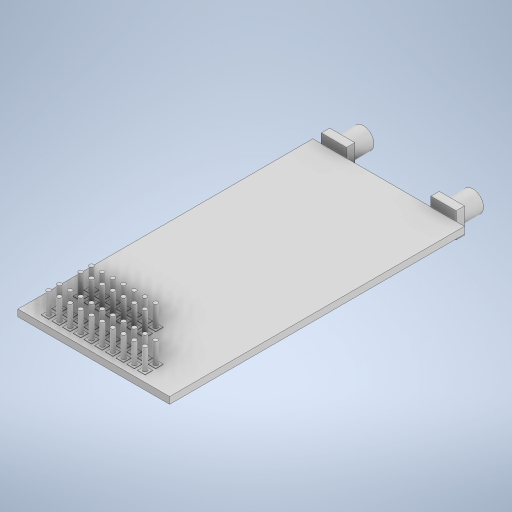
# Autodesk Inventor part: LoRa_board
Saved by Autodesk Inventor 2023 (Build 270158000, 158)
## iProperties
Created: 2023-03-23
Part Number: LoRa_board
Material: 一般
Document SubType Name: Modeling
Designer: 310611102
Density: 1 g/cm^3
Appearance: 預設
Author: 310611102
Autodesk Inventor part; units mm, degrees
ref_plane "YZ Plane" through (0, 0, 0) normal (1, 0, 0) x (0, 1, 0)
ref_plane "XZ Plane" through (0, 0, 0) normal (0, 1, 0) x (-1, 0, 0)
ref_plane "XY Plane" through (0, 0, 0) normal (0, 0, 1) x (1, 0, 0)
sketch "Sketch1" plane through (0, 0, 0) normal (0, 1, 0) x (-1, 0, 0)
  line L0 (18, 35) -> (-18, 35)
  line L1 (-18, 35) -> (-18, -35)
  line L2 (-18, -35) -> (18, -35)
  line L3 (18, -35) -> (18, 35)
  line L4 (18, 35) -> (-18, -35) construction
  line L5 (-18, 35) -> (18, -35) construction
  point P0 (0, 0)
  dimension "d0" = 70
  dimension "d1" = 36
  constraints: 12 end point, 2 midpoint, 2 parallel, 1 horizontal, 1 perpendicular
  measures "d0" distance of L0.end L1.end
  measures "d1" distance of L1.end L2.end
extrude "Extrusion1" add sketch "Sketch1" along normal blind 1.6
sketch "Sketch2" plane through (0, 1.6, 0) normal (0, 1, 0) x (1, 0, 0)
  line L0 (-14, -31.7) -> (-12.2, -31.7)
  line L1 (-12.2, -31.7) -> (-12.2, -33.5)
  line L2 (-12.2, -33.5) -> (-14, -33.5)
  line L3 (-14, -33.5) -> (-14, -31.7)
  line L4 (-14, -31.7) -> (-12.2, -33.5) construction
  line L5 (-12.2, -31.7) -> (-14, -33.5) construction
  line L6 (-11.46, -33.5) -> (-11.46, -31.7)
  line L7 (-11.46, -31.7) -> (-9.66, -31.7)
  line L8 (-9.66, -31.7) -> (-9.66, -33.5)
  line L9 (-9.66, -33.5) -> (-11.46, -33.5)
  line L10 (-8.92, -33.5) -> (-8.92, -31.7)
  line L11 (-8.92, -31.7) -> (-7.12, -31.7)
  line L12 (-7.12, -31.7) -> (-7.12, -33.5)
  line L13 (-7.12, -33.5) -> (-8.92, -33.5)
  line L14 (-6.38, -33.5) -> (-6.38, -31.7)
  line L15 (-6.38, -31.7) -> (-4.58, -31.7)
  line L16 (-4.58, -31.7) -> (-4.58, -33.5)
  line L17 (-4.58, -33.5) -> (-6.38, -33.5)
  line L18 (-3.84, -33.5) -> (-3.84, -31.7)
  line L19 (-3.84, -31.7) -> (-2.04, -31.7)
  line L20 (-2.04, -31.7) -> (-2.04, -33.5)
  line L21 (-2.04, -33.5) -> (-3.84, -33.5)
  line L22 (-1.3, -33.5) -> (-1.3, -31.7)
  line L23 (-1.3, -31.7) -> (0.5, -31.7)
  line L24 (0.5, -31.7) -> (0.5, -33.5)
  line L25 (0.5, -33.5) -> (-1.3, -33.5)
  line L26 (1.24, -33.5) -> (1.24, -31.7)
  line L27 (1.24, -31.7) -> (3.04, -31.7)
  line L28 (3.04, -31.7) -> (3.04, -33.5)
  line L29 (3.04, -33.5) -> (1.24, -33.5)
  line L30 (3.78, -33.5) -> (3.78, -31.7)
  line L31 (3.78, -31.7) -> (5.58, -31.7)
  line L32 (5.58, -31.7) -> (5.58, -33.5)
  line L33 (5.58, -33.5) -> (3.78, -33.5)
  line L34 (6.32, -33.5) -> (6.32, -31.7)
  line L35 (6.32, -31.7) -> (8.12, -31.7)
  line L36 (8.12, -31.7) -> (8.12, -33.5)
  line L37 (8.12, -33.5) -> (6.32, -33.5)
  line L38 (8.86, -33.5) -> (8.86, -31.7)
  line L39 (8.86, -31.7) -> (10.66, -31.7)
  line L40 (10.66, -31.7) -> (10.66, -33.5)
  line L41 (10.66, -33.5) -> (8.86, -33.5)
  line L42 (-14, -30.96) -> (-14, -29.16)
  line L43 (-14, -29.16) -> (-12.2, -29.16)
  line L44 (-12.2, -29.16) -> (-12.2, -30.96)
  line L45 (-12.2, -30.96) -> (-14, -30.96)
  line L46 (-11.46, -30.96) -> (-11.46, -29.16)
  line L47 (-11.46, -29.16) -> (-9.66, -29.16)
  line L48 (-9.66, -29.16) -> (-9.66, -30.96)
  line L49 (-9.66, -30.96) -> (-11.46, -30.96)
  line L50 (-8.92, -30.96) -> (-8.92, -29.16)
  line L51 (-8.92, -29.16) -> (-7.12, -29.16)
  line L52 (-7.12, -29.16) -> (-7.12, -30.96)
  line L53 (-7.12, -30.96) -> (-8.92, -30.96)
  line L54 (-6.38, -30.96) -> (-6.38, -29.16)
  line L55 (-6.38, -29.16) -> (-4.58, -29.16)
  line L56 (-4.58, -29.16) -> (-4.58, -30.96)
  line L57 (-4.58, -30.96) -> (-6.38, -30.96)
  line L58 (-3.84, -30.96) -> (-3.84, -29.16)
  line L59 (-3.84, -29.16) -> (-2.04, -29.16)
  line L60 (-2.04, -29.16) -> (-2.04, -30.96)
  line L61 (-2.04, -30.96) -> (-3.84, -30.96)
  line L62 (-1.3, -30.96) -> (-1.3, -29.16)
  line L63 (-1.3, -29.16) -> (0.5, -29.16)
  line L64 (0.5, -29.16) -> (0.5, -30.96)
  line L65 (0.5, -30.96) -> (-1.3, -30.96)
  line L66 (1.24, -30.96) -> (1.24, -29.16)
  line L67 (1.24, -29.16) -> (3.04, -29.16)
  line L68 (3.04, -29.16) -> (3.04, -30.96)
  line L69 (3.04, -30.96) -> (1.24, -30.96)
  line L70 (3.78, -30.96) -> (3.78, -29.16)
  line L71 (3.78, -29.16) -> (5.58, -29.16)
  line L72 (5.58, -29.16) -> (5.58, -30.96)
  line L73 (5.58, -30.96) -> (3.78, -30.96)
  line L74 (6.32, -30.96) -> (6.32, -29.16)
  line L75 (6.32, -29.16) -> (8.12, -29.16)
  line L76 (8.12, -29.16) -> (8.12, -30.96)
  line L77 (8.12, -30.96) -> (6.32, -30.96)
  line L78 (8.86, -30.96) -> (8.86, -29.16)
  line L79 (8.86, -29.16) -> (10.66, -29.16)
  line L80 (10.66, -29.16) -> (10.66, -30.96)
  line L81 (10.66, -30.96) -> (8.86, -30.96)
  line L82 (-18, 35) -> (-18, -35) projected
  line L83 (-18, -35) -> (18, -35) projected
  line L84 (-14, -24.1) -> (-12.2, -24.1)
  line L85 (-12.2, -24.1) -> (-12.2, -25.9)
  line L86 (-12.2, -25.9) -> (-14, -25.9)
  line L87 (-14, -25.9) -> (-14, -24.1)
  line L88 (-11.46, -25.9) -> (-11.46, -24.1)
  line L89 (-9.66, -25.9) -> (-11.46, -25.9)
  line L90 (-9.66, -24.1) -> (-9.66, -25.9)
  line L91 (-11.46, -24.1) -> (-9.66, -24.1)
  line L92 (-8.92, -25.9) -> (-8.92, -24.1)
  line L93 (-7.12, -25.9) -> (-8.92, -25.9)
  line L94 (-7.12, -24.1) -> (-7.12, -25.9)
  line L95 (-8.92, -24.1) -> (-7.12, -24.1)
  line L96 (-6.38, -25.9) -> (-6.38, -24.1)
  line L97 (-4.58, -25.9) -> (-6.38, -25.9)
  line L98 (-4.58, -24.1) -> (-4.58, -25.9)
  line L99 (-6.38, -24.1) -> (-4.58, -24.1)
  line L100 (-3.84, -25.9) -> (-3.84, -24.1)
  line L101 (-2.04, -25.9) -> (-3.84, -25.9)
  line L102 (-2.04, -24.1) -> (-2.04, -25.9)
  line L103 (-3.84, -24.1) -> (-2.04, -24.1)
  line L104 (-1.3, -25.9) -> (-1.3, -24.1)
  line L105 (0.5, -25.9) -> (-1.3, -25.9)
  line L106 (0.5, -24.1) -> (0.5, -25.9)
  line L107 (-1.3, -24.1) -> (0.5, -24.1)
  line L108 (1.24, -25.9) -> (1.24, -24.1)
  line L109 (3.04, -25.9) -> (1.24, -25.9)
  line L110 (3.04, -24.1) -> (3.04, -25.9)
  line L111 (1.24, -24.1) -> (3.04, -24.1)
  line L112 (-14, -23.36) -> (-14, -21.56)
  line L113 (-12.2, -23.36) -> (-14, -23.36)
  line L114 (-12.2, -21.56) -> (-12.2, -23.36)
  line L115 (-14, -21.56) -> (-12.2, -21.56)
  line L116 (-11.46, -23.36) -> (-11.46, -21.56)
  line L117 (-9.66, -23.36) -> (-11.46, -23.36)
  line L118 (-9.66, -21.56) -> (-9.66, -23.36)
  line L119 (-11.46, -21.56) -> (-9.66, -21.56)
  line L120 (-8.92, -23.36) -> (-8.92, -21.56)
  line L121 (-7.12, -23.36) -> (-8.92, -23.36)
  line L122 (-7.12, -21.56) -> (-7.12, -23.36)
  line L123 (-8.92, -21.56) -> (-7.12, -21.56)
  line L124 (-6.38, -23.36) -> (-6.38, -21.56)
  line L125 (-4.58, -23.36) -> (-6.38, -23.36)
  line L126 (-4.58, -21.56) -> (-4.58, -23.36)
  line L127 (-6.38, -21.56) -> (-4.58, -21.56)
  line L128 (-3.84, -23.36) -> (-3.84, -21.56)
  line L129 (-2.04, -23.36) -> (-3.84, -23.36)
  line L130 (-2.04, -21.56) -> (-2.04, -23.36)
  line L131 (-3.84, -21.56) -> (-2.04, -21.56)
  line L132 (-1.3, -23.36) -> (-1.3, -21.56)
  line L133 (0.5, -23.36) -> (-1.3, -23.36)
  line L134 (0.5, -21.56) -> (0.5, -23.36)
  line L135 (-1.3, -21.56) -> (0.5, -21.56)
  line L136 (1.24, -23.36) -> (1.24, -21.56)
  line L137 (3.04, -23.36) -> (1.24, -23.36)
  line L138 (3.04, -21.56) -> (3.04, -23.36)
  line L139 (1.24, -21.56) -> (3.04, -21.56)
  point P0 (0, 0)
  point P1 (-13.1, -32.6)
  point P2 (-14, -25)
  dimension "d4" = 1.8
  dimension "d5" = 1.8
  dimension "d8" = 2.54
  dimension "d11" = 2.54
  dimension "d14" = 4
  dimension "d15" = 1.5
  dimension "d20" = 1.8
  dimension "d21" = 1.8
  dimension "d24" = 2.54
  dimension "d27" = 2.54
  dimension "d70" = 4
  dimension "d71" = 10
  constraints: 276 end point, 4 collinear, 4 horizontal, 4 parallel, 3 midpoint, 2 perpendicular, 2 vertical, 252 other
  measures "d4" distance of L0.start L0.end
  measures "d5" distance of L0.end L1.end
  measures "d8" distance of L2.end L6.start
  measures "d11" distance of L2.end L42.start
  measures "d14" distance between parallel lines of L82 L3
  measures "d15" distance between parallel lines of L83 L2
  measures "d20" distance of L87.end L84.end
  measures "d21" distance of L84.end L86.start
  measures "d24" distance of L86.end L88.start
  measures "d27" distance of L86.end L112.start
  measures "d70" distance between parallel lines of L82 L87
  measures "d71" distance from line of L83 point (-14, -25)
extrude "Extrusion2" add sketch "Sketch2" along normal blind 0.1 and the other way blind 2
sketch "Sketch4" plane through (0, 1.7, 0) normal (0, 1, 0) x (1, 0, 0)
  circle A0 centre (-13.1, -32.6) radius 0.5
  line L0 (-12.2, -33.5) -> (-12.2, -31.7) projected
  line L1 (-12.2, -31.7) -> (-14, -31.7) projected
  circle A1 centre (-10.56, -32.6) radius 0.5
  circle A2 centre (-8.02, -32.6) radius 0.5
  circle A3 centre (-5.48, -32.6) radius 0.5
  circle A4 centre (-2.94, -32.6) radius 0.5
  circle A5 centre (-0.4, -32.6) radius 0.5
  circle A6 centre (2.14, -32.6) radius 0.5
  circle A7 centre (4.68, -32.6) radius 0.5
  circle A8 centre (7.22, -32.6) radius 0.5
  circle A9 centre (9.76, -32.6) radius 0.5
  circle A10 centre (-13.1, -30.06) radius 0.5
  circle A11 centre (-10.56, -30.06) radius 0.5
  circle A12 centre (-8.02, -30.06) radius 0.5
  circle A13 centre (-5.48, -30.06) radius 0.5
  circle A14 centre (-2.94, -30.06) radius 0.5
  circle A15 centre (-0.4, -30.06) radius 0.5
  circle A16 centre (2.14, -30.06) radius 0.5
  circle A17 centre (4.68, -30.06) radius 0.5
  circle A18 centre (7.22, -30.06) radius 0.5
  circle A19 centre (9.76, -30.06) radius 0.5
  circle A20 centre (-13.1, -25) radius 0.5
  line L2 (-12.2, -24.1) -> (-14, -24.1) projected
  line L3 (-12.2, -25.9) -> (-12.2, -24.1) projected
  circle A21 centre (-10.56, -25) radius 0.5
  circle A22 centre (-8.02, -25) radius 0.5
  circle A23 centre (-5.48, -25) radius 0.5
  circle A24 centre (-2.94, -25) radius 0.5
  circle A25 centre (-0.4, -25) radius 0.5
  circle A26 centre (2.14, -25) radius 0.5
  circle A27 centre (-13.1, -22.46) radius 0.5
  circle A28 centre (-10.56, -22.46) radius 0.5
  circle A29 centre (-8.02, -22.46) radius 0.5
  circle A30 centre (-5.48, -22.46) radius 0.5
  circle A31 centre (-2.94, -22.46) radius 0.5
  circle A32 centre (-0.4, -22.46) radius 0.5
  circle A33 centre (2.14, -22.46) radius 0.5
  point P0 (0, 0)
  point P1 (-12.2, -32.6)
  point P2 (-13.1, -31.7)
  point P3 (-13.1, -24.1)
  point P4 (-12.2, -25)
  dimension "d32" = 1
  dimension "d35" = 2.54
  dimension "d38" = 2.54
  dimension "d45" = 1
  dimension "d48" = 2.54
  dimension "d51" = 2.54
  constraints: 34 centre point, 4 midpoint, 2 horizontal, 2 horizontal alignment, 2 vertical, 2 vertical alignment, 64 other
  measures "d32" diameter of A0
  measures "d35" distance of A0.centre A1.centre
  measures "d38" distance of A0.centre A10.centre
  measures "d45" diameter of A20
  measures "d48" distance of A20.centre A21.centre
  measures "d51" distance of A20.centre A27.centre
extrude "Extrusion3" add sketch "Sketch4" along normal blind 5
sketch "Sketch7" plane through (18, 0, -35) normal (0, 0, -1) x (-1, 0, 0)
  line L0 (8, -2.2) -> (2, -2.2)
  line L1 (2, -2.2) -> (2, 3.8)
  line L2 (2, 3.8) -> (8, 3.8)
  line L3 (8, 3.8) -> (8, -2.2)
  line L4 (8, -2.2) -> (2, 3.8) construction
  line L5 (2, -2.2) -> (8, 3.8) construction
  line L6 (28, -2.2) -> (34, -2.2)
  line L7 (34, -2.2) -> (34, 3.8)
  line L8 (34, 3.8) -> (28, 3.8)
  line L9 (28, 3.8) -> (28, -2.2)
  line L10 (28, -2.2) -> (34, 3.8) construction
  line L11 (34, -2.2) -> (28, 3.8) construction
  line L12 (0, 0) -> (0, 1.6) projected
  line L13 (36, 0) -> (36, 1.6) projected
  point P0 (18, 0)
  point P1 (5, 0.8)
  point P2 (31, 0.8)
  point P3 (0, 0.8)
  dimension "d72" = 6
  dimension "d73" = 6
  dimension "d74" = 6
  dimension "d75" = 6
  dimension "d76" = 5
  dimension "d77" = 5
  constraints: 24 end point, 5 midpoint, 4 parallel, 2 horizontal, 2 perpendicular, 1 horizontal alignment, 1 point on line
  measures "d72" distance of L0.start L0.end
  measures "d73" distance of L0.end L1.end
  measures "d74" distance of L8.end L6.start
  measures "d75" distance of L6.start L6.end
  measures "d76" distance from line of L12 point (5, 0.8)
  measures "d77" distance from line of L13 point (31, 0.8)
extrude "Extrusion6" add sketch "Sketch7" along normal blind 2
sketch "Sketch8" plane through (18, 0, -37) normal (0, 0, -1) x (-1, 0, 0)
  circle A0 centre (5, 0.8) radius 2.5
  circle A1 centre (31, 0.8) radius 2.5
  line L0 (0, 0) -> (0, 1.6) projected
  line L1 (2, -2.2) -> (8, -2.2) projected
  line L2 (28, -2.2) -> (34, -2.2) projected
  point P0 (18, 0)
  point P1 (0, 0.8)
  point P2 (5, -2.2)
  point P3 (31, -2.2)
  dimension "d80" = 5
  dimension "d81" = 5
  constraints: 3 midpoint, 2 centre point, 2 horizontal alignment, 2 vertical alignment
  measures "d80" diameter of A1
  measures "d81" diameter of A0
extrude "Extrusion7" add sketch "Sketch8" along normal blind 5
body "Solid1"
